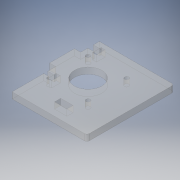
# Autodesk Inventor part: Belt_Holder2
Saved by Autodesk Inventor 2016 (Build 200138000, 138)
## iProperties
Created: 2018-05-31
Part Number: Belt_Holder2
Material: Polycarbonate, Clear
Document SubType Name: Modeling
Designer: Phil Erle
Density: 1.2 g/cm^3
Appearance: Polycarbonate - Clear
Author: Phil Erle
Autodesk Inventor part; units mm, degrees
ref_plane "YZ Plane" through (0, 0, 0) normal (1, 0, 0) x (0, 1, 0)
ref_plane "XZ Plane" through (0, 0, 0) normal (0, 1, 0) x (-1, 0, 0)
ref_plane "XY Plane" through (0, 0, 0) normal (0, 0, 1) x (1, 0, 0)
sketch "Sketch1" plane through (0, 0, 0) normal (0, 0, 1) x (1, 0, 0)
  line L0 (29, 35) -> (-29, 35)
  line L1 (-29, 35) -> (-29, 20)
  line L2 (-29, 20) -> (-34, 20)
  line L3 (-34, 20) -> (-34, 0)
  line L4 (-34, 0) -> (-29, 0)
  line L5 (-29, 0) -> (-29, -35)
  line L6 (-29, -35) -> (29, -35)
  line L7 (31, -33) -> (31, 33)
  arc A0 (31, 33) -> (29, 35) centre (29, 33) ccw
  arc A1 (29, -35) -> (31, -33) centre (29, -33) ccw
  point P0 (0, 0)
  point P1 (31, 35)
  point P2 (31, -35)
  point P3 (31, 0)
  point P4 (0, 35)
  dimension "d0" = 70
  dimension "d1" = 5
  dimension "d2" = 20
  dimension "d3" = 15
  dimension "d4" = 60
  dimension "d7" = 2
  constraints: 16 end point, 6 perpendicular, 6 point on line, 4 point on circle, 4 tangent, 2 centre point, 2 midpoint, 1 equal radius, 1 horizontal, 1 horizontal alignment, 1 vertical alignment
  measures "d0" distance of point (31, -35) point (31, 35)
  measures "d1" distance between parallel lines of L3 L1
  measures "d2" distance of L2.end L3.end
  measures "d3" distance between parallel lines of L0 L2
  measures "d4" distance of point (31, 35) L0.end
  measures "d7" radius of A0
extrude "Extrusion1" add sketch "Sketch1" along normal blind 5
sketch "Sketch2" plane through (0, 0, 5) normal (0, 0, 1) x (1, 0, 0)
  line L0 (-29, 35) -> (-29, 20) projected
  point P0 (0, 0)
  point P1 (-8, 5)
  dimension "d8" = 5
  dimension "d33" = 21
  measures "d8" vertical distance of point (-8, 5) point (0, 0)
  measures "d33" distance from line of L0 point (-8, 5)
hole "Hole1" at (-8, 5, 5) direction (0, 0, -1) diameter 22 depth 8 tip angle 118
sketch "Sketch3" plane through (0, 0, 5) normal (0, 0, 1) x (1, 0, 0)
  circle A0 centre (-8, 5) radius 11 projected
  line L0 (-23.5, -10.5) -> (7.5, -10.5) construction
  line L1 (7.5, -10.5) -> (7.5, 20.5) construction
  line L2 (7.5, 20.5) -> (-23.5, 20.5) construction
  line L3 (-23.5, 20.5) -> (-23.5, -10.5) construction
  line L4 (-23.5, -10.5) -> (7.5, 20.5) construction
  line L5 (7.5, -10.5) -> (-23.5, 20.5) construction
  point P0 (0, 0)
  dimension "d17" = 31
  dimension "d18" = 31
  constraints: 12 end point, 4 coincident, 2 midpoint, 2 parallel, 1 horizontal, 1 perpendicular
  measures "d17" distance of L1.end L2.end
  measures "d18" distance of L0.end L1.end
hole "Hole2" at (-23.5, 20.5, 5) at (7.5, 20.5, 5) at (7.5, -10.5, 5) at (-23.5, -10.5, 5) direction (0, 0, -1) diameter 3.4 depth 8 tip angle 118 clearance for "Countersunk Flat Head Screw DIN EN ISO 2009" size "M3" standard "DIN"
sketch "Sketch4" plane through (0, 0, 5) normal (0, 0, 1) x (1, 0, 0)
  line L0 (-29, 20) -> (-29, 35) projected
  line L1 (-29, 30.25) -> (-24, 30.25)
  line L2 (-24, 30.25) -> (-24, 31.5)
  line L3 (-24, 31.5) -> (-20.8, 31.5)
  line L4 (-20.8, 31.5) -> (-20.8, 24.5)
  line L5 (-20.8, 24.5) -> (-24, 24.5)
  line L6 (-24, 24.5) -> (-24, 25.75)
  line L7 (-24, 25.75) -> (-29, 25.75)
  line L8 (-29, 25.75) -> (-29, 30.25)
  line L9 (-29, 20) -> (-34, 20) projected
  line L10 (-29, -6.4) -> (-24, -6.4)
  line L11 (-24, -6.4) -> (-24, -4.5)
  line L12 (-24, -4.5) -> (-20.8, -4.5)
  line L13 (-20.8, -4.5) -> (-20.8, -11.5)
  line L14 (-20.8, -11.5) -> (-24, -11.5)
  line L15 (-24, -11.5) -> (-24, -9.6)
  line L16 (-24, -9.6) -> (-29, -9.6)
  line L17 (-29, -9.6) -> (-29, -6.4)
  line L18 (-29, -35) -> (-29, 0) projected
  line L19 (-34, 0) -> (-29, 0) projected
  point P0 (0, 0)
  point P1 (-29, 28)
  point P2 (-20.8, 28)
  point P3 (-20.8, -8)
  point P4 (-29, -8)
  dimension "d37" = 7
  dimension "d38" = 3.2
  dimension "d39" = 5
  dimension "d42" = 4.5
  dimension "d43" = 8
  dimension "d44" = 7
  dimension "d45" = 3.2
  dimension "d46" = 5
  dimension "d47" = 3.2
  dimension "d48" = 8
  constraints: 32 end point, 10 perpendicular, 6 point on line, 4 midpoint, 2 collinear, 2 horizontal, 2 horizontal alignment, 1 vertical alignment
  measures "d37" distance of L3.end L4.end
  measures "d38" distance of L2.end L3.end
  measures "d39" distance of L1.start L1.end
  measures "d42" distance between parallel lines of L7 L1
  measures "d43" distance from line of point (-29, 28) L9
  measures "d44" distance of L12.end L13.end
  measures "d45" distance of L11.end L12.end
  measures "d46" distance of L10.start L10.end
  measures "d47" distance between parallel lines of L16 L10
  measures "d48" distance from line of L19 point (-29, -8)
extrude "Extrusion2" cut sketch "Sketch4" against normal blind 5
sketch "Sketch5" plane through (0, 0, 5) normal (0, 0, 1) x (1, 0, 0)
  line L0 (-5, -25) -> (5, -25)
  line L1 (5, -25) -> (5, -20)
  line L2 (5, -20) -> (-5, -20)
  line L3 (-5, -20) -> (-5, -25)
  line L4 (-5, -25) -> (5, -20) construction
  line L5 (5, -25) -> (-5, -20) construction
  line L6 (-29, -35) -> (29, -35) projected
  point P0 (0, 0)
  point P1 (0, -22.5)
  point P2 (0, -22.5)
  dimension "d28" = 10
  dimension "d29" = 5
  dimension "d34" = 10
  constraints: 12 end point, 3 midpoint, 2 parallel, 1 horizontal, 1 perpendicular, 1 vertical alignment
  measures "d28" distance of L2.end L1.end
  measures "d29" distance of L1.end L0.end
  measures "d34" distance between parallel lines of L6 L0
extrude "Extrusion3" cut sketch "Sketch5" against normal blind 5
body "Solid1"
